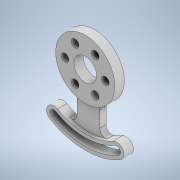
# Autodesk Inventor part: 3.3
Saved by Autodesk Inventor 2020 (Build 240168000, 168)
## iProperties
Created: 2022-03-24
Part Number: 3.3
Material: Типовые
Document SubType Name: Modeling
Designer: guest
Density: 1 g/cm^3
Appearance: По умолчанию
Author: guest
Autodesk Inventor part; units mm, degrees
ref_plane "YZ Plane" through (0, 0, 0) normal (1, 0, 0) x (0, 1, 0)
ref_plane "XZ Plane" through (0, 0, 0) normal (0, 1, 0) x (-1, 0, 0)
ref_plane "XY Plane" through (0, 0, 0) normal (0, 0, 1) x (1, 0, 0)
sketch "Эскиз1" plane through (0, 0, 0) normal (0, 0, 1) x (1, 0, 0)
  circle A0 centre (0, 0) radius 18
  arc A1 (23.0877, -40.9385) -> (-23.0877, -40.9385) centre (0, 0) ccw
  circle A2 centre (0, 0) radius 32
  circle A3 centre (-32, 0) radius 6
  arc A4 (-53, -91.7987) -> (53, -91.7987) centre (0, 0) ccw
  arc A5 (-47, -81.4064) -> (47, -81.4064) centre (0, 0) ccw
  arc A6 (-47, -81.4064) -> (-53, -91.7987) centre (-50, -86.6025) ccw
  arc A7 (53, -91.7987) -> (47, -81.4064) centre (50, -86.6025) ccw
  arc A8 (-55.75, -96.5618) -> (55.75, -96.5618) centre (0, 0) ccw
  arc A9 (-44.25, -76.6432) -> (44.25, -76.6432) centre (0, 0) ccw
  arc A10 (-44.25, -76.6432) -> (-55.75, -96.5618) centre (-50, -86.6025) ccw
  arc A11 (55.75, -96.5618) -> (44.25, -76.6432) centre (50, -86.6025) ccw
  line L0 (18, -49.6488) -> (18, -74.7747)
  line L1 (-18, -49.6488) -> (-18, -74.7747)
  arc A12 (-30.0566, -83.2397) -> (-18, -74.7747) centre (-27, -74.7747) ccw
  arc A13 (18, -74.7747) -> (30.0566, -83.2397) centre (27, -74.7747) ccw
  arc A14 (-23.0877, -40.9385) -> (23.0877, -40.9385) centre (0, 0) ccw
  arc A15 (-18, -49.6488) -> (-23.0877, -40.9385) centre (-28, -49.6488) ccw
  arc A16 (23.0877, -40.9385) -> (18, -49.6488) centre (28, -49.6488) ccw
  line L2 (0, 50.4106) -> (0, -115.4701)
  line L3 (-32, 7.0837) -> (-32, -7.0862)
  line L4 (-38.6315, -0.0012) -> (-25.0914, -0.0012)
  circle A17 centre (-16, -27.7128) radius 6
  line L5 (-19.3147, -33.4565) -> (-12.5446, -21.7304)
  line L6 (-22.1346, -24.171) -> (-9.8632, -31.2559)
  circle A18 centre (16, -27.7128) radius 6
  line L7 (19.3168, -33.4552) -> (12.5468, -21.7292)
  line L8 (9.8654, -31.2547) -> (22.1368, -24.1697)
  circle A19 centre (32, 0) radius 6
  line L9 (38.6315, 0.0012) -> (25.0914, 0.0012)
  line L10 (32, -7.0837) -> (32, 7.0862)
  circle A20 centre (16, 27.7128) radius 6
  line L11 (19.3147, 33.4565) -> (12.5446, 21.7304)
  line L12 (22.1346, 24.171) -> (9.8632, 31.2559)
  circle A21 centre (-16, 27.7128) radius 6
  line L13 (-19.3168, 33.4552) -> (-12.5468, 21.7292)
  line L14 (-9.8654, 31.2547) -> (-22.1368, 24.1697)
  line L15 (-48.8351, 0.0012) -> (48.9386, 0.0012)
  line L16 (0, 0) -> (-58.0184, -100.4908)
  line L17 (0, 0) -> (58.0184, -100.4908)
  arc A22 (0, -100) -> (63.7418, -77.0518) centre (0, 0) ccw
  arc A23 (-63.7418, -77.0518) -> (0, -100) centre (0, 0) ccw
  point P0 (-18, -86.6502)
  point P1 (18, -86.6502)
  dimension "d31" = 64
  dimension "d23" = 360
  dimension "d25" = 11.5
  dimension "d26" = 6
  dimension "d27" = 10
  dimension "d28" = 9
  dimension "d29" = 111.5
  dimension "d30" = 47
  dimension "d32" = 36
  dimension "d33" = 0
  dimension "d34" = 0.0025
  dimension "d35" = 31.7418
  dimension "d36" = 26.0184
  dimension "d37" = 23.75
  dimension "d38" = 16.9386
  dimension "d39" = 6.6315
  dimension "d40" = 7.0849
  dimension "d41" = 0
  dimension "d42" = 7.0849
  dimension "d43" = 6.9086
  dimension "d44" = 50.4094
  dimension "d45" = 115.4713
  dimension "d46" = 76.25
  dimension "d47" = 80.8351
  constraints: 39 point on circle, 36 end point, 23 centre point, 18 tangent, 6 coincident, 4 vertical, 3 equal radius, 3 point on line, 2 horizontal, 2 parallel, 2 symmetric about line, 1 horizontal alignment, 52 other
  measures "d25" radius of A11
  measures "d26" radius of A7
  measures "d27" radius of A16
  measures "d28" radius of A13
  measures "d29" radius of A8
  measures "d30" radius of A14
  measures "d32" diameter of A0
  measures "d33" distance between parallel lines of L15 L9
  measures "d34" distance between parallel lines of L9 L4
  measures "d35" distance from line of A22.end L10
  measures "d36" distance from line of L17.end L10
  measures "d37" distance from line of A8.end L10
  measures "d38" distance from line of L15.end L10
  measures "d39" distance from line of L9.start L10
  measures "d40" distance from line of L10.end L9
  measures "d41" distance from line of A19.centre L10
  measures "d42" distance from line of L10.start L9
  measures "d43" distance from line of L9.end L10
  measures "d44" distance from line of L2.start L9
  measures "d45" distance from line of L2.end L9
  measures "d46" distance from line of A9.start L10
  measures "d47" distance from line of L15.start L10
sketch "Эскиз2" plane through (0, 0, 0) normal (0, 1, 0) x (-1, 0, 0)
  circle A0 centre (0, 0) radius 13
  arc A1 (45, 0) -> (36.8236, 25.8654) centre (0, 0) ccw
  arc A2 (48, 83.1384) -> (-48, 83.1384) centre (0, 0) ccw
  arc A3 (32, 55.4256) -> (-32, 55.4256) centre (0, 0) ccw
  arc A4 (32, 55.4256) -> (48, 83.1384) centre (40, 69.282) ccw
  arc A5 (-48, 83.1384) -> (-32, 55.4256) centre (-40, 69.282) ccw
  arc A6 (54, 93.5307) -> (-54, 93.5307) centre (0, 0) ccw
  arc A7 (-54, 93.5307) -> (-67.9609, 67.8035) centre (-40, 69.282) ccw
  line L0 (-52, 0) -> (52, 0)
  arc A8 (-45, 0) -> (-36.8236, -25.8654) centre (0, 0) ccw
  arc A9 (-67.9609, 67.8035) -> (-43.6891, 41.5261) centre (-40, 69.282) ccw
  line L1 (0, 108) -> (0, -108)
  arc A10 (-47, -81.4064) -> (47, -81.4064) centre (0, 0) ccw
  arc A11 (-33, -57.1577) -> (33, -57.1577) centre (0, 0) ccw
  arc A12 (-33, -57.1577) -> (-47, -81.4064) centre (-40, -69.282) ccw
  arc A13 (47, -81.4064) -> (33, -57.1577) centre (40, -69.282) ccw
  arc A14 (-54, -93.5307) -> (54, -93.5307) centre (0, 0) ccw
  arc A15 (54, -93.5307) -> (43.6891, -41.5261) centre (40, -69.282) ccw
  arc A16 (-43.6891, -41.5261) -> (-36.8236, -25.8654) centre (-45.0067, -31.6133) ccw
  arc A17 (36.8236, -25.8654) -> (43.6891, -41.5261) centre (45.0067, -31.6133) ccw
  arc A18 (36.8236, -25.8654) -> (45, 0) centre (0, 0) ccw
  arc A19 (-43.6891, -41.5261) -> (-54, -93.5307) centre (-40, -69.282) ccw
  arc A20 (-36.8236, 25.8654) -> (-43.6891, 41.5261) centre (-45.0067, 31.6133) ccw
  arc A21 (-36.8236, 25.8654) -> (-45, 0) centre (0, 0) ccw
  arc A22 (43.6891, 41.5261) -> (36.8236, 25.8654) centre (45.0067, 31.6133) ccw
  arc A23 (43.6891, 41.5261) -> (54, 93.5307) centre (40, 69.282) ccw
  line L2 (-41.1412, -18.232) -> (-65.599, 57.9377)
  line L3 (41.1412, -18.232) -> (65.599, 57.9377)
  arc A24 (-61.4245, -51.2545) -> (61.4245, -51.2545) centre (0, 0) ccw
  arc A25 (61.4245, 51.2545) -> (-61.4245, 51.2545) centre (0, 0) ccw
  line L4 (0, 0) -> (-54, -93.5307)
  line L5 (0, 0) -> (54, -93.5307)
  line L6 (0, 0) -> (-54, 93.5307)
  line L7 (0, 0) -> (54, 93.5307)
  arc A26 (-14.56, 37.256) -> (-24.2581, 31.8048) centre (0, 0) ccw construction
  dimension "d48" = 10
  dimension "d49" = 28
  dimension "d50" = 16
  dimension "d51" = 14
  dimension "d52" = 108
  dimension "d53" = 45
  dimension "d54" = 26
  dimension "d56" = 12.198
  dimension "d57" = 47.802
  dimension "d60" = 4.765
  dimension "d61" = 1.8998
  dimension "d62" = 69.9981
  dimension "d63" = 77.5654
  dimension "d65" = 94.2555
  dimension "d66" = 44.7453
  dimension "d67" = 0
  dimension "d68" = 0
  dimension "d84" = 40
  dimension "d85" = 0
  constraints: 65 point on circle, 27 centre point, 18 tangent, 16 end point, 9 point on line, 8 coincident, 7 symmetric about line, 2 collinear, 2 equal radius, 1 perpendicular, 1 vertical, 2 other
  measures "d48" radius of A22
  measures "d49" radius of A23
  measures "d50" radius of A4
  measures "d51" radius of A13
  measures "d52" radius of A6
  measures "d53" radius of A21
  measures "d54" diameter of A0
  measures "d56" angle of L7 L3
  measures "d57" angle of L5 L3
  measures "d60" distance from line of L0.end L3
  measures "d61" distance from line of A1.start L3
  measures "d62" distance from line of A26.start L3
  measures "d63" distance from line of A26.end L3
  measures "d65" distance from line of L0.start L3
  measures "d66" distance from line of point (0, 0) L3
  measures "d67" distance from line of point (0, 0) L7
  measures "d68" distance from line of point (0, 0) L0
  measures "d84" radius of A26
  measures "d85" distance from line of point (0, 0) L5
sketch "Эскиз3" plane through (0, 0, 0) normal (1, 0, 0) x (0, 1, 0)
  line L0 (2, 0) -> (17, 0)
  line L1 (20, -2) -> (20, -8)
  line L2 (18, -10) -> (3.4641, -10)
  line L3 (0, -8) -> (0, -2)
  line L4 (-2, 0) -> (-8, 0)
  line L5 (-10, 2) -> (-10, 8)
  line L6 (-8, 10) -> (-2, 10)
  line L7 (0, 8) -> (0, 2)
  line L8 (20, -8) -> (18, -10)
  line L9 (20, -2) -> (17, 0)
  line L10 (0, -8) -> (3.4641, -10)
  arc A0 (-2, 0) -> (0, 2) centre (-2, 2) ccw
  arc A1 (2, 0) -> (0, -2) centre (2, -2) ccw
  arc A2 (-8, 10) -> (-10, 8) centre (-8, 8) ccw
  line L11 (-2, 10) -> (0, 8)
  line L12 (-10, 2) -> (-8, 0)
  point P0 (0, 0)
  point P1 (20, -10)
  point P2 (20, 0)
  point P3 (0, -10)
  point P4 (-10, 10)
  point P5 (-10, 0)
  point P6 (0, 10)
  dimension "d69" = 20
  dimension "d70" = 10
  dimension "d71" = 10
  dimension "d72" = 10
  dimension "d73" = 2
  dimension "d74" = 2
  dimension "d75" = 2
  dimension "d76" = 3
  dimension "d77" = 2
  dimension "d78" = 60
  dimension "d79" = 2
  dimension "d80" = 2
  dimension "d81" = 45
  dimension "d82" = 2
  dimension "d83" = 45
  constraints: 26 end point, 16 point on line, 6 point on circle, 6 tangent, 4 parallel, 3 centre point, 2 equal radius, 2 horizontal, 2 perpendicular
  measures "d69" distance of point (20, -10) point (0, -10)
  measures "d70" distance of point (20, 0) point (20, -10)
  measures "d71" distance of point (-10, 10) point (0, 10)
  measures "d72" distance of point (-10, 0) point (-10, 10)
  measures "d73" distance of L1.end point (20, -10)
  measures "d74" distance of L2.start point (20, -10)
  measures "d75" distance of L1.start point (20, 0)
  measures "d76" distance of L0.end point (20, 0)
  measures "d77" distance of L3.start point (0, -10)
  measures "d78" angle of L3 L10
  measures "d79" radius of A0
  measures "d80" distance of L6.end point (0, 10)
  measures "d81" angle of L6 L11
  measures "d82" distance of L5.start point (-10, 0)
  measures "d83" angle of L5 L12
extrude "Выдавливание1" add sketch "Эскиз1" along normal blind 10 contours L15 L9 A19 A2 A18 L7 L17 A0 | A0 L2 A2 A20 A19 L9 L15 | A0 L15 A3 A2 A21 L2 | L17 L7 A18 A2 L2 A0 | A0 L16 L5 A17 A2 A3 L15 | L2 A1 L15 L9 A19 A2 A20 | A2 A21 A3 L15 A1 L2 | L2 A2 A17 L5 L16 A0 | L2 A14 A1 L16 L5 A17 A2 | A2 A18 L7 L17 A1 A14 L2 | A19 L9 L15 A1 L17 L7 A18 A2 | A2 A17 L5 L16 A1 L15 A3 | L2 A9 A12 L1 A15 A14 | A14 A16 L0 A13 A9 L2 | L2 A5 L16 A9 | A9 L17 A5 L2 | A11 A22 A7 L17 | L16 A6 A23 A10 | A11 L17 A7 A22 | A23 A6 L16 A10 | A8 L2 A4 L17 | L16 A4 L2 A8
extrude "Выдавливание2" add sketch "Эскиз1" along normal blind 15 contours L15 L9 A19 A2 A18 L7 L17 A0 | A0 L2 A2 A20 A19 L9 L15 | A0 L15 A3 A2 A21 L2 | L17 L7 A18 A2 L2 A0 | A0 L16 L5 A17 A2 A3 L15 | L2 A1 L15 L9 A19 A2 A20 | A2 A21 A3 L15 A1 L2 | L2 A2 A17 L5 L16 A0 | L2 A14 A1 L16 L5 A17 A2 | A2 A18 L7 L17 A1 A14 L2 | A19 L9 L15 A1 L17 L7 A18 A2 | A2 A17 L5 L16 A1 L15 A3 | L2 A5 L16 A9 | A9 L17 A5 L2 | A11 A22 A7 L17 | L16 A6 A23 A10 | A11 L17 A7 A22 | A23 A6 L16 A10 | A8 L2 A4 L17 | L16 A4 L2 A8
equation "\"d74\" = d73"
equation "\"d82\" = d80"
equation "\"d83\" = d81"
